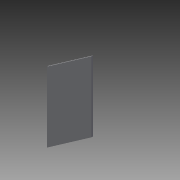
# Autodesk Inventor part: Left Abdomen
Saved by Autodesk Inventor 2014 (Build 180170000, 170)
## iProperties
Created: 2015-08-01
Part Number: Left Abdomen
Material: Generic
Document SubType Name: Modeling
Designer: Devon
Density: 1 g/cm^3
Appearance: Default
Author: Devon
Autodesk Inventor part; units mm, degrees
ref_plane "YZ Plane" through (0, 0, 0) normal (1, 0, 0) x (0, 1, 0)
ref_plane "XZ Plane" through (0, 0, 0) normal (0, 1, 0) x (-1, 0, 0)
ref_plane "XY Plane" through (0, 0, 0) normal (0, 0, 1) x (1, 0, 0)
sketch "Sketch1" plane through (0, 0, 0) normal (0, 0, 1) x (1, 0, 0)
  line L0 (-24.3533, 25.6313) -> (-24.3533, -114.0687)
  line L1 (-24.3533, -114.0687) -> (64.0742, -52.1511)
  line L2 (-24.3533, -114.0687) -> (83.5967, -114.0687) construction
  line L3 (64.0742, -52.1511) -> (64.0742, 87.5489)
  line L4 (64.0742, 87.5489) -> (-24.3533, 25.6313)
  point P0 (0, 0)
  dimension "d0" = 139.7
  dimension "d1" = 107.95
  dimension "d2" = 35
  dimension "d3" = 139.7
  constraints: 10 end point, 1 equal length, 1 horizontal, 1 perpendicular, 1 vertical
  measures "d0" distance of L0.start L0.end
  measures "d1" distance of L0.end L1.end
  measures "d2" angle of L2 L1
  measures "d3" distance of L1.end L3.end
extrude "Extrusion1" add sketch "Sketch1" along normal blind 3.175
sketch "Sketch2" plane through (0, 0, 0) normal (0, 0, -1) x (-1, 0, 0)
  line L0 (21.1783, -44.2187) -> (21.1783, -25.1687)
  line L1 (21.1783, -25.1687) -> (24.3533, -25.1687)
  line L2 (21.1783, -44.2187) -> (21.1783, -63.2687)
  line L3 (21.1783, -63.2687) -> (24.3533, -63.2687)
  line L4 (24.3533, -25.1687) -> (24.3533, -63.2687)
  point P0 (0, 0)
  dimension "d7" = 19.05
  dimension "d8" = 19.05
  constraints: 10 end point, 2 perpendicular
  measures "d7" distance of L0.start L0.end
  measures "d8" distance of L0.start L2.end
extrude "Extrusion2" add sketch "Sketch2" along normal blind 79.2734
sketch "Sketch3" plane through (-24.3533, -114.0687, 3.175) normal (-1, 0, 0) x (0, 0, 1)
  line L0 (-82.4484, 88.9) -> (-63.3984, 88.9)
  line L1 (-63.3984, 88.9) -> (-63.3984, 69.85)
  line L2 (-63.3984, 69.85) -> (-82.4484, 69.85)
  line L3 (-82.4484, 69.85) -> (-82.4484, 88.9)
  point P0 (-3.175, 114.0687)
  dimension "d11" = 19.05
  dimension "d12" = 19.05
  constraints: 8 end point, 2 parallel, 1 horizontal, 1 perpendicular
  measures "d11" distance of L1.end L2.end
  measures "d12" distance of L0.end L1.end
hole "Hole1" at (-24.3533, -44.2187, -60.2234) direction (1, 0, 0) diameter 8.3312 end through all
body "Solid1"
